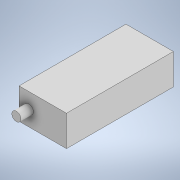
# Autodesk Inventor part: Power brick
Saved by Autodesk Inventor 2022 (Build 260153000, 153)
## iProperties
Created: 2021-12-02
Part Number: Power brick
Material: Generic
Document SubType Name: Modeling
Designer: efred
Density: 1 g/cm^3
Appearance: Default
Author: efred
Autodesk Inventor part; units mm, degrees
ref_plane "YZ Plane" through (0, 0, 0) normal (1, 0, 0) x (0, 1, 0)
ref_plane "XZ Plane" through (0, 0, 0) normal (0, 1, 0) x (-1, 0, 0)
ref_plane "XY Plane" through (0, 0, 0) normal (0, 0, 1) x (1, 0, 0)
sketch "Sketch1" plane through (0, 0, 0) normal (0, 1, 0) x (-1, 0, 0)
  line L0 (-25.5, 57.5) -> (25.5, 57.5)
  line L1 (25.5, 57.5) -> (25.5, -57.5)
  line L2 (25.5, -57.5) -> (-25.5, -57.5)
  line L3 (-25.5, -57.5) -> (-25.5, 57.5)
  line L4 (-25.5, 57.5) -> (25.5, -57.5) construction
  line L5 (25.5, 57.5) -> (-25.5, -57.5) construction
  point P0 (0, 0)
  dimension "d0" = 51
  dimension "d1" = 115
  constraints: 12 end point, 2 midpoint, 2 parallel, 1 horizontal, 1 perpendicular
  measures "d0" distance of L0.start L0.end
  measures "d1" distance of L0.end L1.end
extrude "Extrusion1" add sketch "Sketch1" along normal blind 33
sketch "Sketch2" plane through (-25.5, 0, 57.5) normal (0, 0, 1) x (1, 0, 0)
  circle A0 centre (10.5, 16.5) radius 4.875
  line L0 (0, 0) -> (0, 33) projected
  point P0 (25.5, 0)
  point P1 (0, 16.5)
  dimension "d4" = 10.5
  dimension "d5" = 9.75
  constraints: 1 centre point, 1 horizontal alignment, 1 midpoint
  measures "d4" distance from line of L0 A0.centre
  measures "d5" diameter of A0
extrude "Extrusion2" add sketch "Sketch2" along normal blind 13.4
body "Solid1"
